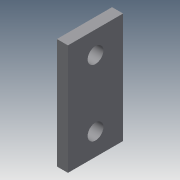
# Autodesk Inventor part: block
Saved by Autodesk Inventor 2015 (Build 190159000, 159)
## iProperties
Created: 2014-08-30
Part Number: block
Material: Generic
Document SubType Name: Modeling
Designer: shohei
Density: 1 g/cm^3
Appearance: Default
Author: shohei
Autodesk Inventor part; units mm, degrees
ref_plane "YZ Plane" through (0, 0, 0) normal (1, 0, 0) x (0, 1, 0)
ref_plane "XZ Plane" through (0, 0, 0) normal (0, 1, 0) x (-1, 0, 0)
ref_plane "XY Plane" through (0, 0, 0) normal (0, 0, 1) x (1, 0, 0)
sketch "Sketch1" plane through (0, 0, 0) normal (1, 0, 0) x (0, 1, 0)
  line L0 (0, 0) -> (50, 0)
  line L1 (50, 0) -> (50, 100)
  line L2 (50, 100) -> (0, 100)
  line L3 (0, 100) -> (0, 0)
  line L4 (25, 108.4087) -> (25, -21.5037)
  circle A0 centre (25, 80) radius 7.1359
  line L5 (63.0593, 50) -> (-7.0373, 50)
  circle A1 centre (25, 20) radius 7.1359
  dimension "d0" = 100
  dimension "d1" = 50
  dimension "d4" = 25
  dimension "d5" = 20
  dimension "d6" = 50
  constraints: 12 end point, 2 centre point, 2 horizontal, 2 parallel, 1 perpendicular, 1 point on line, 1 symmetric about line, 1 vertical, 1 other
  measures "d0" distance of L0.end L1.end
  measures "d1" distance of L1.end L2.end
  measures "d4" distance between parallel lines of L3 L4
  measures "d5" distance from line of L2 A0.centre
  measures "d6" distance between parallel lines of L2 L5
extrude "Extrusion2" add sketch "Sketch1" along normal blind 10 contours L3 L5 L4 A1 L0 | L4 A1 L5 L1 L0 | L3 L2 L4 A0 L5 | L4 A0 L2 L1 L5
equation "\"d4\" = 0.5 * d1"
equation "\"d5\" = 0.2 * d0"
equation "\"d6\" = 0.5 * d0"
body "Solid2"
